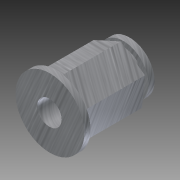
# Autodesk Inventor part: Hub
Saved by Autodesk Inventor 2012 (Build 160160000, 160)
## iProperties
Created: 2012-03-02
Part Number: Hub
Material: Default
Document SubType Name: Modeling
Designer: Lauszus
Density: 1 g/cm^3
Author: Lauszus
Autodesk Inventor part; units mm, degrees
ref_plane "YZ Plane" through (0, 0, 0) normal (1, 0, 0) x (0, 1, 0)
ref_plane "XZ Plane" through (0, 0, 0) normal (0, 1, 0) x (-1, 0, 0)
ref_plane "XY Plane" through (0, 0, 0) normal (0, 0, 1) x (1, 0, 0)
sketch "Sketch1" plane through (0, 0, 0) normal (0, 0, 1) x (1, 0, 0)
  line L0 (-6.5322, -3.0499) -> (-5.8184, 4.2476) projected
  line L1 (-5.8184, 4.2476) -> (0.8584, 7.2782) projected
  line L2 (0.8584, 7.2782) -> (6.8213, 3.0112) projected
  line L3 (6.8213, 3.0112) -> (6.1075, -4.2863) projected
  line L4 (6.1075, -4.2863) -> (-0.5693, -7.3169) projected
  line L5 (-0.5693, -7.3169) -> (-6.5322, -3.0499) projected
  circle A0 centre (0.1445, -0.0193) radius 15.5 projected
  line L6 (-6.7574, 4.9196) -> (-7.5837, -3.5272)
  line L7 (-7.5837, -3.5272) -> (-0.6817, -8.4661)
  line L8 (-0.6817, -8.4661) -> (7.0465, -4.9582)
  line L9 (7.0465, -4.9582) -> (7.8727, 3.4885)
  line L10 (7.8727, 3.4885) -> (0.9708, 8.4274)
  line L11 (0.9708, 8.4274) -> (-6.7574, 4.9196)
  circle A1 centre (0.1445, -0.0193) radius 8.487
  point P0 (0, 0)
  dimension "d0" = 1
  constraints: 12 end point, 1 coincident, 8 other
  measures "d0" distance between parallel lines of L0 L6
extrude "Extrusion1" add sketch "Sketch1" along normal blind 1.5 contours L0 L1 L2 L3 L4 L5 | L11 L10 L9 L8 L7 L6 | A1 L11 | L6 A1 | L7 A1 | A1 L10 | L8 A1 | A1 L9
sketch "Sketch2" plane through (0, 0, 0) normal (0, 0, -1) x (-1, 0, 0)
  line L0 (5.8184, 4.2476) -> (6.5322, -3.0499) projected
  line L1 (6.5322, -3.0499) -> (0.5693, -7.3169) projected
  line L2 (0.5693, -7.3169) -> (-6.1075, -4.2863) projected
  line L3 (-6.1075, -4.2863) -> (-6.8213, 3.0112) projected
  line L4 (-6.8213, 3.0112) -> (-0.8584, 7.2782) projected
  line L5 (-0.8584, 7.2782) -> (5.8184, 4.2476) projected
  circle A0 centre (-0.1445, -0.0193) radius 15.5 projected
  line L6 (5.8184, 4.2476) -> (6.5322, -3.0499) projected
  line L7 (6.5322, -3.0499) -> (0.5693, -7.3169) projected
  line L8 (0.5693, -7.3169) -> (-6.1075, -4.2863) projected
  line L9 (-6.1075, -4.2863) -> (-6.8213, 3.0112) projected
  line L10 (-6.8213, 3.0112) -> (-0.8584, 7.2782) projected
  line L11 (-0.8584, 7.2782) -> (5.8184, 4.2476) projected
  circle A1 centre (-0.1445, -0.0193) radius 15.5 projected
  point P0 (0, 0)
extrude "Extrusion2" add sketch "Sketch2" along normal blind 18.24 contours L0 L1 L2 L3 L4 L5
ref_plane "Work Plane1" through (0, 0, -15.24) normal (0, 0, -1) x (-1, 0, 0)
sketch "Sketch3" plane through (0, 0, -15.24) normal (0, 0, -1) x (-1, 0, 0)
  line L0 (5.8184, 4.2476) -> (6.5322, -3.0499) projected
  line L1 (-0.8584, 7.2782) -> (5.8184, 4.2476) projected
  line L2 (-6.8213, 3.0112) -> (-0.8584, 7.2782) projected
  line L3 (-6.1075, -4.2863) -> (-6.8213, 3.0112) projected
  line L4 (0.5693, -7.3169) -> (-6.1075, -4.2863) projected
  line L5 (6.5322, -3.0499) -> (0.5693, -7.3169) projected
  circle A0 centre (0, 0) radius 4.9486
  dimension "d17" = 9.8971
  constraints: 1 centre point, 1 coincident
  measures "d17" diameter of A0
sketch "Sketch4" plane through (0, 0, 1.5) normal (0, 0, 1) x (1, 0, 0)
  circle A0 centre (0, 0) radius 3
  dimension "d8" = 6
  constraints: 1 centre point, 1 coincident
  measures "d8" diameter of A0
extrude "Extrusion4" cut sketch "Sketch4" against normal through all
extrude "Extrusion6" cut sketch "Sketch3" along normal blind 1.5
sketch "Sketch6" plane through (0, 0, -18.24) normal (0, 0, -1) x (-1, 0, 0)
  circle A0 centre (0, 0) radius 3 projected
  line L0 (5.8184, 4.2476) -> (6.5322, -3.0499) projected
  line L1 (-0.8584, 7.2782) -> (5.8184, 4.2476) projected
  line L2 (-6.8213, 3.0112) -> (-0.8584, 7.2782) projected
  line L3 (-6.1075, -4.2863) -> (-6.8213, 3.0112) projected
  line L4 (0.5693, -7.3169) -> (-6.1075, -4.2863) projected
  line L5 (6.5322, -3.0499) -> (0.5693, -7.3169) projected
  circle A1 centre (0, 0) radius 6.2043
  constraints: 1 centre point, 1 coincident, 1 tangent
extrude "Extrusion7" cut sketch "Sketch6" against normal up to surface (1.5 mm away)
body "Solid1"
